safety pin v2 (Autodesk Fusion 360 design; units mm, degrees)
Autodesk Fusion 360 part; units mm, degrees
sketch "Sketch1" plane through (0, 0, 0) normal (0, 0, 1) x (1, 0, 0)
  line L0 (0, 0) -> (0, 50)
  line L1 (0, 50) -> (30, 50) construction
  line L2 (30, 50) -> (30, -50)
  line L3 (30, -50) -> (10, -50) construction
  line L4 (10, -50) -> (10, 35)
  line L5 (10, 35) -> (23.6636, 35) construction
  line L6 (23.6636, 35) -> (23.6636, -35)
  line L7 (23.6636, -35) -> (18.6636, -35) construction
  arc A0 (30, 50) -> (0, 50) centre (15, 50) ccw
  arc A1 (23.6636, 35) -> (10, 35) centre (16.8318, 35) ccw
  arc A2 (10, -50) -> (30, -50) centre (20, -50) ccw
  arc A3 (18.6636, -35) -> (23.6636, -35) centre (21.1636, -35) ccw
  dimension "d1" = 50
  dimension "d2" = 30
  dimension "d3" = 100
  dimension "d4" = 20
  dimension "d5" = 70
  dimension "d6" = 5
  dimension "d7" = 15
  dimension "d8" = 6.3364
  constraint coincident L0.start origin
  constraint vertical L0
  constraint perpendicular L0 L1
  constraint perpendicular L1 L2
  constraint perpendicular L2 L3
  constraint perpendicular L3 L4
  constraint perpendicular L4 L5
  constraint perpendicular L5 L6
  constraint perpendicular L6 L7
  constraint tangent L0 A0
  constraint tangent L4 A1
  constraint tangent L4 A2
  constraint tangent L6 A3
  measures "d1" distance of L0.start L0.end
  measures "d2" distance of L0.end L1.end
  measures "d3" distance of L1.end L2.end
  measures "d4" distance of L2.end L3.end
  measures "d5" distance of L5.end L6.end
  measures "d6" distance of L6.end L7.end
  measures "d7" distance of L1 L5
  measures "d8" distance of L2 L6
sketch "Sketch2" plane through (0, 0, 0) normal (0, 1, 0) x (1, 0, 0)
sketch "Sketch3" plane through (0, 0, 0) normal (0, 1, 0) x (1, 0, 0)
sketch "Sketch4" plane through (0, 0, 0) normal (0, 1, 0) x (1, 0, 0)
  circle A0 centre (0, 0) radius 0.75
  dimension "d9" = 1.5
  constraint coincident A0.centre origin
  measures "d9" diameter of A0
sweep "Sweep1" add profiles "Sketch4" path "Sketch1" along L0 A0 L2 A2 L4 A1 L6 A3 section 1
